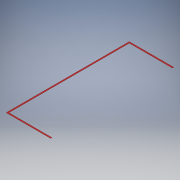
# Autodesk Inventor part: Trim_Red
Saved by Autodesk Inventor 2017.1 (Build 211199000, 199)
## iProperties
Created: 2017-01-05
Part Number: Trim_Red
Material: Generic
Document SubType Name: Modeling
Designer: PhillipD
Density: 1 g/cm^3
Appearance: Smooth - Red
Author: PhillipD
Autodesk Inventor part; units mm, degrees
ref_plane "YZ Plane" through (0, 0, 0) normal (1, 0, 0) x (0, 1, 0)
ref_plane "XZ Plane" through (0, 0, 0) normal (0, 1, 0) x (-1, 0, 0)
ref_plane "XY Plane" through (0, 0, 0) normal (0, 0, 1) x (1, 0, 0)
sketch "Sketch1" plane through (0, 0, 0) normal (0, 1, 0) x (-1, 0, 0)
  line L0 (0, 0) -> (2286, 0)
  line L1 (2286, 0) -> (2286, -6350)
  line L2 (2286, -6350) -> (0, -6350)
  line L3 (0, -6299.2) -> (2235.2, -6299.2)
  line L4 (2235.2, -6299.2) -> (2235.2, -50.8)
  line L5 (2235.2, -50.8) -> (0, -50.8)
  line L6 (0, 0) -> (0, -50.8)
  line L7 (0, -6299.2) -> (0, -6350)
  dimension "d0" = 2286
  dimension "d1" = 6350
  dimension "d2" = 2286
  dimension "d3" = 50.8
  constraints: 16 end point, 4 perpendicular, 1 collinear, 1 horizontal, 1 vertical, 2 other
  measures "d0" distance of L0.start L0.end
  measures "d1" distance of L0.end L1.end
  measures "d2" distance of L1.end L2.end
  measures "d3" distance between parallel lines of L1 L4
extrude "Extrusion1" add sketch "Sketch1" along normal blind 6.35
body "Solid1"
